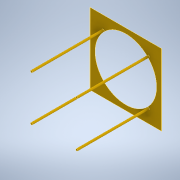
# Autodesk Inventor part: electrode_holder
Saved by Autodesk Inventor 2021 (Build 250183000, 183)
## iProperties
Created: 2020-07-14
Part Number: electrode_holder
Material: Generic
Document SubType Name: Modeling
Designer: aydan
Density: 1 g/cm^3
Appearance: Gold
Author: aydan
Autodesk Inventor part; units mm, degrees
ref_plane "YZ Plane" through (0, 0, 0) normal (1, 0, 0) x (0, 1, 0)
ref_plane "XZ Plane" through (0, 0, 0) normal (0, 1, 0) x (-1, 0, 0)
ref_plane "XY Plane" through (0, 0, 0) normal (0, 0, 1) x (1, 0, 0)
sketch "Sketch1" plane through (0, 0, 0) normal (0, 0, 1) x (1, 0, 0)
  line L0 (-35, 35) -> (35, 35)
  line L1 (35, 35) -> (35, -35)
  line L2 (35, -35) -> (-35, -35)
  line L3 (-35, -35) -> (-35, 35)
  line L4 (-35, 35) -> (35, -35) construction
  line L5 (35, 35) -> (-35, -35) construction
  circle A0 centre (0, 0) radius 30
  dimension "d0" = 70
  dimension "d1" = 70
  dimension "d2" = 60
  constraints: 12 end point, 2 midpoint, 2 parallel, 1 centre point, 1 coincident, 1 horizontal, 1 perpendicular
  measures "d0" distance of L1.end L2.end
  measures "d1" distance of L0.end L1.end
  measures "d2" diameter of A0
extrude "Extrusion1" add sketch "Sketch1" along normal blind 0.1
sketch "Sketch2" plane through (0, 0, 0.1) normal (0, 0, 1) x (1, 0, 0)
  circle A0 centre (-22.097, 22.097) radius 1
  circle A1 centre (22.097, 22.097) radius 1
  circle A2 centre (22.097, -22.097) radius 1
  circle A3 centre (-22.097, -22.097) radius 1
  line L0 (-35, 35) -> (-35, -35) projected
  line L1 (35, 35) -> (-35, 35) projected
  line L2 (35, -35) -> (35, 35) projected
  line L3 (-35, -35) -> (35, -35) projected
  point P0 (0, 0)
  dimension "d5" = 2
  dimension "d6" = 2
  dimension "d7" = 2
  dimension "d8" = 2
  dimension "d9" = 12.903
  dimension "d10" = 12.903
  dimension "d11" = 12.903
  dimension "d12" = 12.903
  dimension "d13" = 12.903
  dimension "d14" = 12.903
  dimension "d15" = 12.903
  dimension "d16" = 12.903
  constraints: 4 centre point
  measures "d5" diameter of A0
  measures "d6" diameter of A1
  measures "d7" diameter of A2
  measures "d8" diameter of A3
  measures "d9" distance from line of L0 A0.centre
  measures "d10" distance from line of A0.centre L1
  measures "d11" distance from line of L1 A1.centre
  measures "d12" distance from line of L2 A1.centre
  measures "d13" distance from line of L2 A2.centre
  measures "d14" distance from line of L3 A2.centre
  measures "d15" distance from line of L3 A3.centre
  measures "d16" distance from line of L0 A3.centre
extrude "Extrusion2" add sketch "Sketch2" along normal blind 70 contours A0 | A1 | A2 | A3
body "Solid1"
